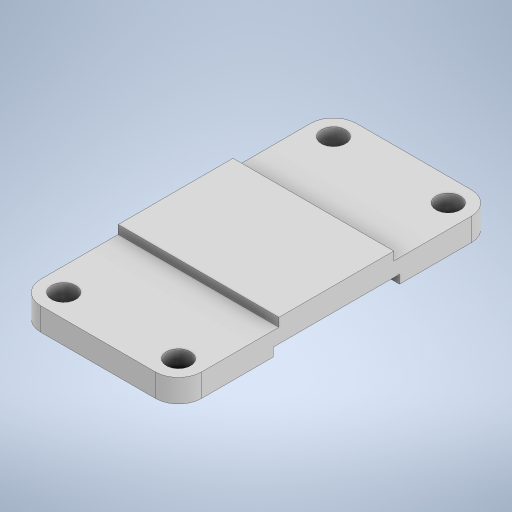
# Autodesk Inventor part: Base polea
Saved by Autodesk Inventor 2024 (Build 280153000, 153)
## iProperties
Created: 2024-03-03
Part Number: Base polea
Material: Genérico
Document SubType Name: Modeling
Designer: kelly
Density: 1 g/cm^3
Appearance: Valor por defecto
Author: kelly
Autodesk Inventor part; units mm, degrees
ref_plane "YZ Plane" through (0, 0, 0) normal (1, 0, 0) x (0, 1, 0)
ref_plane "XZ Plane" through (0, 0, 0) normal (0, 1, 0) x (-1, 0, 0)
ref_plane "XY Plane" through (0, 0, 0) normal (0, 0, 1) x (1, 0, 0)
sketch "Boceto1" plane through (0, 0, 0) normal (0, 1, 0) x (-1, 0, 0)
  line L0 (-20, 55) -> (20, 55)
  line L1 (28, 47) -> (28, -47)
  line L2 (20, -55) -> (-20, -55)
  line L3 (-28, -47) -> (-28, 47)
  line L4 (-28, 55) -> (28, -55) construction
  line L5 (28, 55) -> (-28, -55) construction
  arc A0 (28, 47) -> (20, 55) centre (20, 47) ccw
  arc A1 (20, -55) -> (28, -47) centre (20, -47) ccw
  arc A2 (-28, -47) -> (-20, -55) centre (-20, -47) ccw
  arc A3 (-20, 55) -> (-28, 47) centre (-20, 47) ccw
  circle A4 centre (20, 47) radius 4.25
  circle A5 centre (-20, 47) radius 4.25
  circle A6 centre (20, -47) radius 4.25
  circle A7 centre (-20, -47) radius 4.25
  line L6 (-28, 20) -> (28, 20)
  line L7 (28, 20) -> (28, -20)
  line L8 (28, -20) -> (-28, -20)
  line L9 (-28, -20) -> (-28, 20)
  line L10 (-28, 20) -> (28, -20) construction
  line L11 (28, 20) -> (-28, -20) construction
  point P0 (0, 0)
  dimension "d0" = 56
  dimension "d1" = 110
  dimension "d2" = 8
  dimension "d3" = 8.5
  dimension "d4" = 8.5
  dimension "d5" = 8.5
  dimension "d6" = 8.5
  dimension "d7" = 56
  dimension "d8" = 40
  constraints: 24 end point, 8 centre point, 8 point on circle, 8 point on line, 8 tangent, 4 coincident, 4 midpoint, 4 parallel, 3 equal radius, 2 horizontal, 2 perpendicular
  measures "d0" distance of L4.end L5.end
  measures "d1" distance of L5.start L4.end
  measures "d2" radius of A0
  measures "d3" diameter of A4
  measures "d4" diameter of A5
  measures "d5" diameter of A6
  measures "d6" diameter of A7
  measures "d7" distance of L7.end L8.end
  measures "d8" distance of L6.end L7.end
extrude "Extrusión1" add sketch "Boceto1" along normal blind 8 contours L0 A0 L1 L6 L3 A3 | L8 L1 A1 L2 A2 L3
extrude "Extrusión2" add sketch "Boceto1" along normal blind 11 contours L6 L1 L8 L3
sketch "Boceto2" plane through (28, 0, 47) normal (1, 0, 0) x (0, 0, -1)
  line L0 (25, 3) -> (69, 3)
  line L1 (69, 3) -> (69, 0)
  line L2 (69, 0) -> (25, 0)
  line L3 (25, 0) -> (25, 3)
  line L4 (0, 0) -> (94, 0) projected
  point P0 (47, 0)
  point P1 (47, 0)
  dimension "d13" = 44
  dimension "d14" = 3
  constraints: 8 end point, 2 midpoint, 2 parallel, 1 horizontal, 1 perpendicular
  measures "d13" distance of L1.end L2.end
  measures "d14" distance of L0.end L1.end
extrude "Extrusión3" cut sketch "Boceto2" against normal through all
